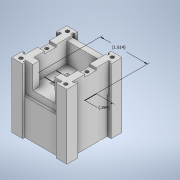
# Autodesk Inventor part: Motor_Holder
Saved by Autodesk Inventor 2022 (Build 260153000, 153)
## iProperties
Created: 2023-02-28
Part Number: Motor_Holder
Material: Generic
Document SubType Name: Modeling
Designer: zarek
Density: 1 g/cm^3
Appearance: Default
Author: zarek
Autodesk Inventor part; units mm, degrees
ref_plane "YZ Plane" through (0, 0, 0) normal (1, 0, 0) x (0, 1, 0)
ref_plane "XZ Plane" through (0, 0, 0) normal (0, 1, 0) x (-1, 0, 0)
ref_plane "XY Plane" through (0, 0, 0) normal (0, 0, 1) x (1, 0, 0)
sketch "Sketch1" plane through (0, 0, 0) normal (0, 1, 0) x (-1, 0, 0)
  line L0 (101.6, 101.6) -> (-101.6, 101.6)
  line L1 (-101.6, 101.6) -> (-101.6, -101.6)
  line L2 (-101.6, -101.6) -> (101.6, -101.6)
  line L3 (101.6, -101.6) -> (101.6, 101.6)
  circle A0 centre (0, 0) radius 2.5
  line L4 (9.525, -6.5) -> (-9.525, -6.5)
  line L5 (0, 0) -> (0, 8)
  line L6 (-14.5, -6.5) -> (-14.5, 22.5)
  line L7 (14.5, 22.5) -> (14.5, -6.5)
  circle A1 centre (0, 8) radius 14
  line L8 (-14.5, 22.5) -> (14.5, 22.5)
  line L9 (14.5, -6.5) -> (-14.5, -6.5)
  line L10 (-24.5, 32.5) -> (24.5, 32.5)
  line L11 (24.5, 32.5) -> (24.5, -16.5)
  line L12 (24.5, -16.5) -> (-24.5, -16.5)
  line L13 (-24.5, -16.5) -> (-24.5, 32.5)
  line L14 (-9.525, 22.5) -> (9.525, 22.5)
  line L15 (9.525, 22.5) -> (9.525, 27.58)
  line L16 (9.525, 27.58) -> (-9.525, 27.58)
  line L17 (-9.525, 27.58) -> (-9.525, 22.5)
  point P0 (9.525, 22.5)
  point P1 (-9.525, -6.5)
  dimension "d0" = 203.2
  dimension "d1" = 203.2
  dimension "d2" = 8
  dimension "d3" = 28
  dimension "d4" = 29
  dimension "d5" = 29
  dimension "d6" = 14.5
  dimension "d7" = 10
  dimension "d8" = 10
  dimension "d9" = 10
  dimension "d10" = 10
  dimension "d11" = 5.08
  dimension "d12" = 9.525
  dimension "d13" = 9.525
  dimension "d14" = 101.6
  dimension "d15" = 101.6
  constraints: 36 end point, 8 parallel, 4 perpendicular, 2 centre point, 2 coincident, 2 point on line, 1 horizontal
  measures "d0" distance between parallel lines of L2 L0
  measures "d1" distance between parallel lines of L1 L3
  measures "d2" distance of L5.start L5.end
  measures "d3" diameter of A1
  measures "d4" distance between parallel lines of L9 L8
  measures "d5" distance between parallel lines of L7 L6
  measures "d6" distance from line of A1.centre L8
  measures "d7" distance between parallel lines of L11 L7
  measures "d8" distance between parallel lines of L8 L10
  measures "d9" distance between parallel lines of L13 L6
  measures "d10" distance between parallel lines of L12 L9
  measures "d11" distance between parallel lines of L14 L16
  measures "d12" distance from line of A1.centre L15
  measures "d13" distance from line of L5.end L17
  measures "d14" distance from line of point (0, 0) L1
  measures "d15" distance from line of L0 point (0, 0)
extrude "Extrusion1" add sketch "Sketch1" along normal blind 56.5 contours A0 | L4 L9 L6 L8 L7 | L8 L17 L16 L15 | A1 | L10 L11 L12 L13
sketch "Sketch2" plane through (0, 56.5, 0) normal (0, 1, 0) x (1, 0, 0)
  line L0 (101.6, 101.6) -> (-101.6, 101.6)
  line L1 (-101.6, 101.6) -> (-101.6, -101.6)
  line L2 (-101.6, -101.6) -> (101.6, -101.6)
  line L3 (101.6, -101.6) -> (101.6, 101.6)
  circle A0 centre (0, 0) radius 2.5
  line L4 (-9.525, 6.5) -> (9.525, 6.5)
  line L5 (0, 0) -> (0, -8)
  line L6 (14.5, 6.5) -> (14.5, -22.5)
  line L7 (-14.5, -22.5) -> (-14.5, 6.5)
  circle A1 centre (0, -8) radius 14
  line L8 (14.5, -22.5) -> (-14.5, -22.5)
  line L9 (-14.5, 6.5) -> (14.5, 6.5)
  line L10 (24.5, -32.5) -> (-24.5, -32.5)
  line L11 (-24.5, -32.5) -> (-24.5, 16.5)
  line L12 (-24.5, 16.5) -> (24.5, 16.5)
  line L13 (24.5, 16.5) -> (24.5, -32.5)
  line L14 (9.525, -22.5) -> (-9.525, -22.5)
  line L15 (-9.525, -22.5) -> (-9.525, -27.58)
  line L16 (-9.525, -27.58) -> (9.525, -27.58)
  line L17 (9.525, -27.58) -> (9.525, -22.5)
  point P0 (9.525, 22.5)
  point P1 (-9.525, -6.5)
  dimension "d18" = 203.2
  dimension "d19" = 203.2
  dimension "d20" = 8
  dimension "d21" = 28
  dimension "d22" = 29
  dimension "d23" = 29
  dimension "d24" = 14.5
  dimension "d25" = 10
  dimension "d26" = 10
  dimension "d27" = 10
  dimension "d28" = 10
  dimension "d29" = 5.08
  dimension "d30" = 9.525
  dimension "d31" = 9.525
  dimension "d32" = 101.6
  dimension "d33" = 101.6
  constraints: 36 end point, 8 parallel, 4 perpendicular, 2 centre point, 2 coincident, 2 point on line, 1 horizontal
  measures "d18" distance between parallel lines of L2 L0
  measures "d19" distance between parallel lines of L1 L3
  measures "d20" distance of L5.start L5.end
  measures "d21" diameter of A1
  measures "d22" distance between parallel lines of L9 L8
  measures "d23" distance between parallel lines of L7 L6
  measures "d24" distance from line of A1.centre L8
  measures "d25" distance between parallel lines of L11 L7
  measures "d26" distance between parallel lines of L8 L10
  measures "d27" distance between parallel lines of L13 L6
  measures "d28" distance between parallel lines of L12 L9
  measures "d29" distance between parallel lines of L14 L16
  measures "d30" distance from line of A1.centre L15
  measures "d31" distance from line of L5.end L17
  measures "d32" distance from line of point (0, 0) L1
  measures "d33" distance from line of L0 point (0, 0)
extrude "Extrusion2" cut sketch "Sketch2" against normal blind 19.5 contours A0 | L4 L9 L6 L8 L7 | L8 L17 L16 L15 | A1
sketch "Sketch4" plane through (0, 56.5, 0) normal (0, 1, 0) x (1, 0, 0)
  circle A0 centre (-17.508, -8) radius 2
  circle A1 centre (17.4854, -8) radius 2
  circle A2 centre (17.4854, -8) radius 2
  circle A3 centre (0, -8.01) radius 14
  circle A4 centre (0, -0.01) radius 2.5
  circle A5 centre (-19.4934, 12.0285) radius 2.2448
  circle A6 centre (19.5, 12.0285) radius 2.3104
  circle A7 centre (19.5, -28.5182) radius 2.2008
  circle A8 centre (-19.4934, -28.5182) radius 2.3894
  point P0 (0, 0)
  dimension "d37" = 34.9934
  dimension "d38" = 28
  dimension "d39" = 8
  dimension "d65" = 8
  dimension "d66" = 8
  constraints: 9 centre point, 2 coincident
  measures "d37" distance of A2.centre A0.centre
  measures "d38" diameter of A3
  measures "d39" distance of point (0, -8.01) A4.centre
  measures "d65" vertical distance of point (0, 0) A2.centre
  measures "d66" vertical distance of A0.centre point (0, 0)
hole "Hole1" at (-17.508, 56.5, 8) at (17.4854, 56.5, 8) at (-19.4934, 56.5, 28.5182) at (19.5, 56.5, 28.5182) at (-19.4934, 56.5, -12.0285) at (19.5, 56.5, -12.0285) direction (0, -1, 0) diameter 2.85 depth 12.7 tip angle 118 countersink diameter 3.0226 countersink angle 82 thread size "M3.5x0.6" class "6H" standard "ANSI Metric M Profile"
sketch "Sketch5" plane through (0, 0, 0) normal (0, -1, 0) x (1, 0, 0)
  circle A0 centre (-19.4934, 28.5182) radius 1.425 projected
  circle A1 centre (-19.4934, 28.5182) radius 1.425
  circle A2 centre (19.5, 28.5182) radius 1.425 projected
  circle A3 centre (19.5, 28.5182) radius 1.425
  circle A4 centre (19.5, -12.0285) radius 1.425 projected
  circle A5 centre (19.5, -12.0285) radius 1.425
  circle A6 centre (-19.4934, -12.0285) radius 1.5113 projected
  circle A7 centre (-19.4934, -12.0285) radius 1.5113
  point P0 (0, 0)
  constraints: 4 centre point, 4 coincident
hole "Hole2" at (19.5, 0, -12.0285) at (-19.4934, 0, -12.0285) at (-19.4934, 0, 28.5182) at (19.5, 0, 28.5182) direction (0, 1, 0) diameter 2.85 depth 12.7 tip angle 118 countersink diameter 3.0226 countersink angle 82 thread size "M3.5x0.6" class "6H" standard "ANSI Metric M Profile"
sketch "Sketch6" plane through (-24.5, 0, 32.5) normal (0, 0, 1) x (1, 0, 0)
  line L0 (34.025, 56.5) -> (34.025, 37) projected
  line L1 (14.975, 56.5) -> (34.025, 56.5)
  line L2 (34.025, 56.5) -> (34.025, 46.75)
  line L3 (34.025, 46.75) -> (14.975, 46.75)
  line L4 (14.975, 46.75) -> (14.975, 56.5)
  point P0 (24.5, 0)
  constraints: 8 end point, 2 parallel, 1 horizontal, 1 midpoint, 1 perpendicular
extrude "Extrusion3" cut sketch "Sketch6" against normal blind 25.4
sketch "Sketch8" plane through (0, 56.5, 0) normal (0, 1, 0) x (1, 0, 0)
  line L0 (-24.5, -3) -> (24.5, -3)
  line L1 (24.5, -3) -> (24.5, -13)
  line L2 (24.5, -13) -> (-24.5, -13)
  line L3 (-24.5, -13) -> (-24.5, -3)
  line L4 (14.5, 6.5) -> (14.5, -22.5) projected
  line L5 (14.5, -3) -> (14.5, -13)
  line L6 (-14.5, -22.5) -> (-14.5, 6.5) projected
  line L7 (-14.5, -3) -> (-14.5, -13)
  line L8 (24.5, -32.5) -> (24.5, 16.5) projected
  line L9 (-24.5, 16.5) -> (-24.5, -32.5) projected
  point P0 (0, 0)
  dimension "d58" = 10
  dimension "d60" = 0
  dimension "d61" = 0
  dimension "d62" = 3
  constraints: 12 end point, 8 point on line, 2 parallel, 1 horizontal, 1 perpendicular
  measures "d58" distance between parallel lines of L2 L0
  measures "d60" distance between parallel lines of L8 L1
  measures "d61" distance between parallel lines of L9 L3
  measures "d62" distance from line of L0 point (0, 0)
extrude "Extrusion4" cut sketch "Sketch8" against normal blind 2 contours L0 L6 L2 L3 | L0 L1 L2 L4
sketch "Sketch9" plane through (0, 56.5, 0) normal (0, 1, 0) x (1, 0, 0)
  line L0 (-14.5, 6.5) -> (14.5, 6.5) projected
  line L1 (24.5, 16.5) -> (-24.5, 16.5) projected
  line L2 (-14.5, 6.5) -> (14.5, 6.5)
  line L3 (14.5, 6.5) -> (14.5, 16.5)
  line L4 (14.5, 16.5) -> (-14.5, 16.5)
  line L5 (-14.5, 16.5) -> (-14.5, 6.5)
  line L6 (14.5, 6.5) -> (14.5, -3) projected
  line L7 (-14.5, 11.5) -> (14.5, 11.5)
  line L8 (-24.5, 16.5) -> (-24.5, -32.5) projected
  line L9 (-14.5, 6.5) -> (-24.5, 6.5)
  line L10 (-24.5, 6.5) -> (-24.5, -22.5)
  line L11 (-24.5, -22.5) -> (-14.5, -22.5)
  line L12 (-14.5, -22.5) -> (-14.5, 6.5)
  line L13 (-9.525, -22.5) -> (-14.5, -22.5) projected
  line L14 (-20.5, 6.5) -> (-20.5, -22.5)
  line L15 (24.5, -32.5) -> (24.5, 16.5) projected
  line L16 (24.5, -22.5) -> (20.5, -22.5)
  line L17 (20.5, -22.5) -> (20.5, 6.5)
  line L18 (20.5, 6.5) -> (24.5, 6.5)
  line L19 (24.5, 6.5) -> (24.5, -22.5)
  line L20 (-24.5, -32.5) -> (24.5, -32.5) projected
  line L21 (14.5, -32.5) -> (14.5, -30.08)
  line L22 (14.5, -30.08) -> (-14.5, -30.08)
  line L23 (-14.5, -30.08) -> (-14.5, -32.5)
  line L24 (-9.525, -27.58) -> (9.525, -27.58) projected
  point P0 (0, 0)
  point P1 (-14.5, 16.5)
  dimension "d67" = 0
  dimension "d68" = 5
  dimension "d69" = 0
  dimension "d71" = 4
  dimension "d72" = 4
  dimension "d98" = 2.5
  constraints: 34 end point, 7 point on line, 6 parallel, 6 perpendicular, 3 horizontal, 2 midpoint, 1 vertical
  measures "d67" distance between parallel lines of L6 L3
  measures "d68" distance between parallel lines of L0 L7
  measures "d69" distance between parallel lines of L13 L11
  measures "d71" distance between parallel lines of L10 L14
  measures "d72" distance between parallel lines of L15 L17
  measures "d98" distance between parallel lines of L22 L24
extrude "Extrusion5" cut sketch "Sketch9" against normal through all contours L5 L1 L3 L7 | L14 L11 L8 L9 | L15 L16 L17 L18 | L23 L22 L21 L20
sketch "Sketch11" plane through (0, 37, 0) normal (0, 1, 0) x (1, 0, 0)
  line L0 (-20.5, -3) -> (-14.5, -3) projected
  line L1 (20.5, -13) -> (20.5, -3) projected
  line L2 (-20.5, -3) -> (20.5, -3)
  line L3 (20.5, -3) -> (20.5, -13)
  line L4 (20.5, -13) -> (-20.5, -13)
  line L5 (-20.5, -13) -> (-20.5, -3)
  point P0 (0, 0)
  dimension "d75" = 41
  dimension "d76" = 10
  constraints: 8 end point, 2 parallel, 1 horizontal, 1 perpendicular
  measures "d75" distance of L1.start L4.end
  measures "d76" distance between parallel lines of L4 L2
sketch "Sketch12" plane through (14.5, 56.5, -11.5) normal (0, 0, -1) x (-1, 0, 0)
  line L0 (0, 0) -> (-6, 0) projected
  line L1 (29, 0) -> (29, -19.5) projected
  line L2 (0, 0) -> (29, 0)
  line L3 (29, 0) -> (29, -2)
  line L4 (29, -2) -> (0, -2)
  line L5 (0, -2) -> (0, 0)
  point P0 (14.5, -56.5)
  dimension "d77" = 2
  constraints: 8 end point, 2 parallel, 1 horizontal, 1 perpendicular, 1 point on line
  measures "d77" distance between parallel lines of L4 L2
extrude "Extrusion6" cut sketch "Sketch12" against normal blind 25.4
sketch "Sketch13" plane through (0, 37, 0) normal (0, 1, 0) x (1, 0, 0)
  line L0 (0, 0) -> (7.62, 0)
  line L1 (7.62, 0) -> (7.62, -15.24)
  line L2 (7.62, -15.24) -> (0, -15.24)
  line L3 (0, -15.24) -> (0, 0)
  line L4 (0, 0) -> (-7.62, 0)
  line L5 (-7.62, 0) -> (-7.62, -15.24)
  line L6 (-7.62, -15.24) -> (0, -15.24)
  line L7 (0, -15.24) -> (0, 0)
  line L8 (14.5, 6.5) -> (-14.5, 6.5) projected
  line L9 (-9.525, -27.58) -> (9.525, -27.58) projected
  dimension "d80" = 7.62
  dimension "d81" = 15.24
  dimension "d82" = 7.62
  dimension "d86" = 15.24
  constraints: 16 end point, 4 parallel, 2 horizontal, 2 perpendicular
  measures "d80" distance of L1.end L2.end
  measures "d81" distance of L0.end L1.end
  measures "d82" distance of L6.end L5.end
  measures "d86" distance between parallel lines of L6 L4
extrude "Extrusion7" cut sketch "Sketch13" against normal through all
sketch "Sketch14" plane through (0, 56.5, 0) normal (0, 1, 0) x (1, 0, 0)
  line L0 (-14.5, 16.5) -> (-24.5, 16.5) projected
  line L1 (24.5, 6.5) -> (24.5, 16.5) projected
  line L2 (-24.5, 16.5) -> (24.5, 16.5)
  line L3 (24.5, 16.5) -> (24.5, 16)
  line L4 (24.5, 16) -> (-24.5, 16)
  line L5 (-24.5, 16) -> (-24.5, 16.5)
  line L6 (24.5, 16.5) -> (14.5, 16.5) projected
  line L7 (9.525, -32.5) -> (24.5, -32.5) projected
  line L8 (24.5, 16.5) -> (24, 16.5)
  line L9 (24, 16.5) -> (24, -32.5)
  line L10 (24, -32.5) -> (24.5, -32.5)
  line L11 (24.5, -32.5) -> (24.5, 16.5)
  line L12 (-24.5, -22.5) -> (-24.5, -32.5) projected
  line L13 (24.5, -32.5) -> (-24.5, -32.5)
  line L14 (-24.5, -32.5) -> (-24.5, -32)
  line L15 (-24.5, -32) -> (24.5, -32)
  line L16 (24.5, -32) -> (24.5, -32.5)
  line L17 (-24.5, -32.5) -> (-9.525, -32.5) projected
  line L18 (-24.5, -32.5) -> (-24, -32.5)
  line L19 (-24, -32.5) -> (-24, 16.5)
  line L20 (-24, 16.5) -> (-24.5, 16.5)
  line L21 (-24.5, 16.5) -> (-24.5, -32.5)
  point P0 (0, 0)
  point P1 (-24.5, 16)
  point P2 (24, 16)
  point P3 (24, -32)
  point P4 (-24, -32)
  point P5 (-24, 16)
  dimension "d89" = 0.5
  dimension "d90" = 0.5
  dimension "d91" = 0.5
  dimension "d92" = 0.5
  constraints: 32 end point, 8 parallel, 4 horizontal, 4 perpendicular, 4 point on line
  measures "d89" distance between parallel lines of L4 L2
  measures "d90" distance of L10.end L9.end
  measures "d91" distance of L13.end L14.end
  measures "d92" distance of L20.end L19.end
extrude "Extrusion8" cut sketch "Sketch14" against normal through all contours L2 L9 L4 L19 L0 | L19 L4 L5 L0 | L19 L15 L12 L21 L4 | L2 L1 L4 L9 | L4 L1 L11 L15 L9 | L19 L13 L12 L15 | L15 L9 L7 L13 L19 | L15 L11 L7 L9
sketch "Sketch18" plane through (0, 56.5, 0) normal (0, 1, 0) x (1, 0, 0)
  line L0 (-20.5, -22.5) -> (-20.5, 6.5) projected
  line L1 (-24, -22.5) -> (-20.5, -22.5) projected
  line L2 (-20.5, 6.5) -> (-22.5, 6.5)
  line L3 (-22.5, 6.5) -> (-22.5, -22.5)
  line L4 (-22.5, -22.5) -> (-20.5, -22.5)
  line L5 (-20.5, -22.5) -> (-20.5, 6.5)
  line L6 (-20.5, 6.5) -> (-22.5, 6.5)
  line L7 (-22.5, 6.5) -> (-22.5, 8)
  line L8 (-22.5, 8) -> (-20.5, 8)
  line L9 (-20.5, 8) -> (-20.5, 6.5)
  line L10 (-20.5, -22.5) -> (-22.5, -22.5)
  line L11 (-22.5, -22.5) -> (-22.5, -24)
  line L12 (-22.5, -24) -> (-20.5, -24)
  line L13 (-20.5, -24) -> (-20.5, -22.5)
  line L14 (-14.5, 16) -> (-14.5, 11.5) projected
  line L15 (14.5, 16) -> (14.5, -3) projected
  line L16 (-14.5, 11.5) -> (14.5, 11.5)
  line L17 (14.5, 11.5) -> (14.5, 13.5)
  line L18 (14.5, 13.5) -> (-14.5, 13.5)
  line L19 (-14.5, 13.5) -> (-14.5, 11.5)
  line L20 (14.5, 13.5) -> (16, 13.5)
  line L21 (16, 13.5) -> (16, 11.5)
  line L22 (16, 11.5) -> (14.5, 11.5)
  line L23 (14.5, 11.5) -> (14.5, 13.5)
  line L24 (-14.5, 13.5) -> (-16, 13.5)
  line L25 (-16, 13.5) -> (-16, 11.5)
  line L26 (-16, 11.5) -> (-14.5, 11.5)
  line L27 (-14.5, 11.5) -> (-14.5, 13.5)
  line L28 (20.5, -3) -> (20.5, 6.5) projected
  line L29 (20.5, -22.5) -> (24, -22.5) projected
  line L30 (20.5, 6.5) -> (22.5, 6.5)
  line L31 (22.5, 6.5) -> (22.5, -22.5)
  line L32 (22.5, -22.5) -> (20.5, -22.5)
  line L33 (20.5, -22.5) -> (20.5, 6.5)
  line L34 (20.5, 6.5) -> (22.5, 6.5)
  line L35 (22.5, 6.5) -> (22.5, 8)
  line L36 (22.5, 8) -> (20.5, 8)
  line L37 (20.5, 8) -> (20.5, 6.5)
  line L38 (20.5, -22.5) -> (22.5, -22.5)
  line L39 (22.5, -22.5) -> (22.5, -24)
  line L40 (22.5, -24) -> (20.5, -24)
  line L41 (20.5, -24) -> (20.5, -22.5)
  line L42 (-14.5, -30.08) -> (14.5, -30.08)
  line L43 (14.5, -30.08) -> (14.5, -28.08)
  line L44 (14.5, -28.08) -> (-14.5, -28.08)
  line L45 (-14.5, -28.08) -> (-14.5, -30.08)
  line L46 (14.5, -28.08) -> (16, -28.08)
  line L47 (16, -28.08) -> (16, -30.08)
  line L48 (16, -30.08) -> (14.5, -30.08)
  line L49 (14.5, -30.08) -> (14.5, -28.08)
  line L50 (-14.5, -28.08) -> (-16, -28.08)
  line L51 (-16, -28.08) -> (-16, -30.08)
  line L52 (-16, -30.08) -> (-14.5, -30.08)
  line L53 (-14.5, -30.08) -> (-14.5, -28.08)
  point P0 (0, 0)
  point P1 (14.5, 11.5)
  dimension "d99" = 2
  dimension "d100" = 1.5
  dimension "d101" = 2
  dimension "d102" = 2
  dimension "d103" = 1.5
  dimension "d104" = 1.5
  dimension "d105" = 2
  dimension "d106" = 1.5
  dimension "d107" = 1.5
  dimension "d108" = 2
  dimension "d109" = 1.5
  dimension "d110" = 1.5
  dimension "d115" = 1.5
  constraints: 96 end point, 24 parallel, 12 horizontal, 12 perpendicular, 9 point on line
  measures "d99" distance of L4.end L3.end
  measures "d100" distance of L6.end L7.end
  measures "d101" distance of L12.end L11.end
  measures "d102" distance of L17.end L16.end
  measures "d103" distance of L21.end L22.end
  measures "d104" distance of L26.end L25.end
  measures "d105" distance of L31.end L32.end
  measures "d106" distance of L35.end L34.end
  measures "d107" distance of L38.end L39.end
  measures "d108" distance of L43.end L42.end
  measures "d109" distance of L47.end L48.end
  measures "d110" distance of L52.end L51.end
  measures "d115" distance between parallel lines of L12 L4
extrude "Extrusion9" cut sketch "Sketch18" against normal blind 25.4
sketch "Sketch19" plane through (-16, 56.5, 28.08) normal (0, 0, 1) x (1, 0, 0)
  line L0 (6.475, -9.75) -> (25.525, -9.75) projected
  line L1 (1.5, -19.5) -> (30.5, -19.5) projected
  line L2 (6.475, -9.75) -> (26.0764, -9.75)
  line L3 (26.0764, -9.75) -> (26.0764, -19.5)
  line L4 (26.0764, -19.5) -> (6.475, -19.5)
  line L5 (6.475, -19.5) -> (6.475, -9.75)
  point P0 (16, -56.5)
  point P1 (6.475, -19.5)
  constraints: 8 end point, 2 parallel, 1 horizontal, 1 perpendicular, 1 point on line
extrude "Extrusion10" cut sketch "Sketch19" against normal blind 25.4
sketch "Sketch20" plane through (20.5, 54.5, 3) normal (1, 0, 0) x (0, 0, -1)
  point P0 (3, -54.5)
equation "\"d86\" = d81"
equation "\"d100\" = d115"
equation "\"d103\" = d115"
equation "\"d104\" = d115"
equation "\"d106\" = d115"
equation "\"d107\" = d115"
equation "\"d109\" = d115"
equation "\"d110\" = d115"
body "Solid1"
